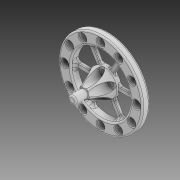
# Autodesk Inventor part: Flywheel
Saved by Autodesk Inventor 2020 (Build 240168000, 168)
## iProperties
Created: 2020-12-31
Part Number: Flywheel
Material: Generic
Document SubType Name: Modeling
Designer: DDeGo
Density: 1 g/cm^3
Appearance: Default
Author: DDeGo
Autodesk Inventor part; units mm, degrees
ref_plane "YZ Plane" through (0, 0, 0) normal (1, 0, 0) x (0, 1, 0)
ref_plane "XZ Plane" through (0, 0, 0) normal (0, 1, 0) x (-1, 0, 0)
ref_plane "XY Plane" through (0, 0, 0) normal (0, 0, 1) x (1, 0, 0)
sketch "Sketch2" plane through (0, 0, 0) normal (0, 0, 1) x (1, 0, 0)
  circle A0 centre (0, 0) radius 1.55
  circle A1 centre (0, 0) radius 9
  dimension "d46" = 18
  dimension "d47" = 3.1
  constraints: 2 centre point, 1 coincident
  measures "d46" diameter of A1
  measures "d47" diameter of A0
extrude "Extrusion2" add sketch "Sketch2" along normal blind 3
sketch "Sketch6" plane through (0, 0, 0) normal (0, 0, -1) x (-1, 0, 0)
  circle A0 centre (0, 0) radius 20
  circle A1 centre (0, 0) radius 28
  dimension "d23" = 56
  dimension "d24" = 8
  constraints: 2 centre point, 2 coincident
  measures "d23" diameter of A1
  measures "d24" radial gap between concentric circles of A0 A1
extrude "Extrusion6" add sketch "Sketch6" against normal blind 5
sketch "Sketch7" plane through (0, 0, 0) normal (0, 0, -1) x (-1, 0, 0)
  line L0 (-3.138, 8.4352) -> (-8.6728, 18.0217)
  circle A0 centre (0, 0) radius 20 projected
  line L1 (-8.6728, 18.0217) -> (-11.2709, 16.5217) construction
  line L2 (-11.2709, 16.5217) -> (-5.7361, 6.9352)
  line L3 (-5.7361, 6.9352) -> (-3.138, 8.4352) construction
  line L4 (0, 0) -> (0, 9) construction
  circle A1 centre (0, 0) radius 9 projected
  point P0 (-3.138, 8.4352)
  dimension "d28" = 3
  dimension "d48" = 30
  constraints: 10 end point, 4 point on circle, 3 perpendicular, 1 vertical
  measures "d28" distance between parallel lines of L0 L2
  measures "d48" angle of L0 L4
extrude "Extrusion7" add sketch "Sketch7" against normal blind 2 contours A1 L2 A0 L0 picked at (-6.1832, 11.0432)
fillet "Fillet1" radius 2 5 edges at (8.6728, 18.0217, 1) (11.2709, 16.5217, 1) (10, 17.3205, 2) (5.7361, 6.9352, 1) (3.138, 8.4352, 1)
fillet "Fillet1" radius 0.5 2 edges at (8.5035, 11.7285, 2) (5.9054, 13.2285, 2)
pattern_circular "Circular Pattern1" count 6 over 360 about axis through (0, 0, 0) along (0, 0, 1) of "Extrusion7", "Fillet1"
sketch "Sketch8" plane through (0, 0, 5) normal (0, 0, 1) x (1, 0, 0)
  circle A0 centre (0, 0) radius 28 projected
  line L0 (28, 0) -> (20, 0) construction
  circle A1 centre (24, 0) radius 2.5
  circle A2 centre (0, 0) radius 20 projected
  dimension "d37" = 5
  constraints: 2 end point, 2 horizontal alignment, 1 centre point, 1 horizontal, 1 midpoint, 1 point on line, 2 other
  measures "d37" diameter of A1
extrude "Extrusion8" cut sketch "Sketch8" against normal through all contours A1
chamfer "Chamfer1" distance 0.5 angle 45 1 edges at (21.5, 0, 5)
pattern_circular "Circular Pattern2" count 12 over 360 about axis through (0, 0, 0) along (0, 0, 1) of "Extrusion8", "Chamfer1"
fillet "Fillet2" radius 1 3 edges at (20, 0, 5) (28, 0, 5) (28, 0, 0)
sketch "Sketch10" plane through (0, 0, 0) normal (0, 0, -1) x (-1, 0, 0)
  circle A0 centre (0, 0) radius 2.6
  dimension "d53" = 5.2
  constraints: 1 centre point, 1 coincident
  measures "d53" diameter of A0
extrude "Extrusion10" cut sketch "Sketch10" against normal blind 2
sketch "Sketch11" plane through (0, 0, 3) normal (0, 0, 1) x (1, 0, 0)
  circle A0 centre (0, 0) radius 3
  dimension "d56" = 6
  constraints: 1 centre point, 1 coincident
  measures "d56" diameter of A0
extrude "Extrusion11" cut sketch "Sketch11" against normal blind 4
sketch "Sketch12" plane through (0, 0, 3) normal (0, 0, 1) x (1, 0, 0)
  line L0 (0, 9) -> (0, 3) construction
  line L1 (0, 0) -> (0, 3) construction
  circle A0 centre (0, 6) radius 1.35
  circle A1 centre (-5.7063, 1.8541) radius 1.35
  circle A2 centre (-3.5267, -4.8541) radius 1.35
  circle A3 centre (3.5267, -4.8541) radius 1.35
  circle A4 centre (5.7063, 1.8541) radius 1.35
  circle A5 centre (0, 0) radius 6 construction
  circle A6 centre (0, 0) radius 3 construction
  point P0 (10, 0)
  point P1 (10, 0)
  dimension "d69" = 12
  dimension "d62" = 2.7
  dimension "d65" = 360
  constraints: 5 centre point, 4 end point, 2 coincident, 2 vertical alignment, 1 collinear, 1 midpoint, 1 vertical, 13 other
  measures "d62" diameter of A0
extrude "Extrusion12" cut sketch "Sketch12" against normal through all
sketch "Sketch16" plane through (0, 0, 0) normal (0, 1, 0) x (-1, 0, 0)
  line L0 (-3, 3) -> (3, 3) projected
  line L1 (9, 3) -> (-9, 3) projected
  line L2 (0, 3) -> (0, 24)
  line L3 (9, 3) -> (3.6, 16)
  line L4 (2.6, 16) -> (2.6, 24)
  line L5 (2.6, 24) -> (0, 24)
  line L6 (3.6, 16) -> (2.6, 16)
  point P0 (0, 0)
  dimension "d75" = 2.6
  dimension "d76" = 8
  dimension "d77" = 13
  dimension "d83" = 1
  constraints: 10 end point, 2 vertical, 1 horizontal, 1 midpoint, 1 perpendicular
  measures "d75" distance between parallel lines of L4 L2
  measures "d76" distance of L4.start L4.end
  measures "d77" distance from line of L1 L4.start
  measures "d83" distance of L3.end L4.start
revolve "Revolution1" add sketch "Sketch16" angle 360 about axis through (0, 0, 3) along (0, 0, 1)
sketch "Sketch15" plane through (0, 0, 0) normal (0, 0, -1) x (-1, 0, 0)
  circle A0 centre (0, 0) radius 4.1
  dimension "d72" = 8.2
  constraints: 1 centre point, 1 coincident
  measures "d72" diameter of A0
extrude "Extrusion14" cut sketch "Sketch15" against normal blind 2
sketch "Sketch17" plane through (-3.5267, -4.8541, 3) normal (0, 0, -1) x (-1, 0, 0)
  circle A0 centre (2.1796, 6.7082) radius 1.35 construction
  circle A1 centre (0, 0) radius 1.35 construction
  circle A2 centre (-7.0534, 0) radius 1.35 construction
  circle A3 centre (-9.2331, 6.7082) radius 1.35 construction
  circle A4 centre (-3.5267, 10.8541) radius 1.35 construction
  circle A5 centre (2.1796, 6.7082) radius 3
  circle A6 centre (-3.5267, 10.8541) radius 3
  circle A7 centre (-9.2331, 6.7082) radius 3
  circle A8 centre (-7.0534, 0) radius 3
  circle A9 centre (0, 0) radius 3
  point P0 (-3.5267, 4.8541)
  dimension "d79" = 6
  constraints: 5 centre point, 5 coincident, 4 equal radius
  measures "d79" diameter of A9
extrude "Extrusion15" cut sketch "Sketch17" against normal through all
fillet "Fillet3" radius 1 1 edges at (2.6, 0, 24)
body "Solid2"
